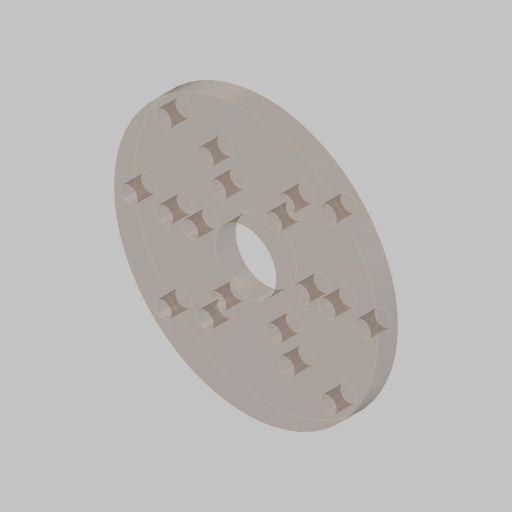
# Autodesk Inventor part: GP9-003
Saved by Autodesk Inventor 2023.5 (Build 275446000, 446)
## iProperties
Created: 2025-02-24
Part Number: GP9-003
Material: Polycarbonate, Smoke
Document SubType Name: Modeling
Designer: dlangdon
Density: 1.2 g/cm^3
Appearance: Polycarbonate - Smoked
Author: dlangdon
Autodesk Inventor part; units mm, degrees
ref_plane "YZ Plane" through (0, 0, 0) normal (1, 0, 0) x (0, 1, 0)
ref_plane "XZ Plane" through (0, 0, 0) normal (0, 1, 0) x (-1, 0, 0)
ref_plane "XY Plane" through (0, 0, 0) normal (0, 0, 1) x (1, 0, 0)
sketch "Sketch1" plane through (0, 0, 0) normal (0, 0, 1) x (1, 0, 0)
  circle A0 centre (0, 0) radius 9.525
  circle A1 centre (0, 0) radius 31.75 construction
  circle A2 centre (-36.5125, 0) radius 4.7625 construction
  circle A3 centre (36.5125, 0) radius 4.7625 construction
  circle A4 centre (0, 0) radius 17.4625 construction
  line L0 (-36.5125, 0) -> (36.5125, 0) construction
  circle A5 centre (0, 0) radius 25.4 construction
  circle A6 centre (0, 0) radius 36.5125 construction
  line L1 (0, 36.5125) -> (0, 0) construction
  line L2 (-25.8182, 25.8182) -> (0, 0) construction
  circle A7 centre (-25.8182, 25.8182) radius 4.7625 construction
  circle A8 centre (-25.8182, -25.8182) radius 4.7625 construction
  circle A9 centre (25.8182, -25.8182) radius 4.7625 construction
  circle A10 centre (25.8182, 25.8182) radius 4.7625 construction
  circle A11 centre (0, 0) radius 41.275
  point P0 (-17.4625, 0)
  point P1 (-25.4, 0)
  point P2 (-12.7, -21.997)
  point P3 (-8.7313, -15.123)
  point P4 (12.7, -21.997)
  point P5 (8.7312, -15.123)
  point P6 (25.4, 0)
  point P7 (17.4625, 0)
  point P8 (12.7, 21.997)
  point P9 (8.7313, 15.123)
  point P10 (-12.7, 21.997)
  point P11 (-8.7312, 15.123)
  dimension "d3" = 34.925
  dimension "d18" = 50.8
  dimension "d0" = 19.05
  dimension "d1" = 63.5
  dimension "d2" = 9.525
  dimension "d21" = 360
  dimension "d30" = 45
  dimension "d33" = 360
  dimension "d37" = 360
  constraints: 12 coincident, 10 centre point, 6 end point, 5 horizontal alignment, 3 point on circle, 2 equal radius, 1 horizontal, 1 midpoint, 1 point on line, 1 tangent, 1 vertical, 31 other
  measures "d0" diameter of A0
  measures "d1" diameter of A1
  measures "d2" diameter of A2
  measures "d30" angle of L1 L2
extrude "Extrusion1" add sketch "Sketch1" along normal blind 6.35
hole "Hole2" at (-17.4625, 0, 0) at (-36.5125, 0, 0) at (36.5125, 0, 0) at (-25.4, 0, 0) at (-12.7, -21.997, 0) at (-8.7313, -15.123, 0) at (12.7, -21.997, 0) at (8.7312, -15.123, 0) at (25.4, 0, 0) at (17.4625, 0, 0) at (12.7, 21.997, 0) at (8.7313, 15.123, 0) at (-12.7, 21.997, 0) at (-8.7312, 15.123, 0) at (-25.8182, 25.8182, 0) at (25.8182, 25.8182, 0) at (25.8182, -25.8182, 0) at (-25.8182, -25.8182, 0) direction (0, 0, 1) diameter 5.1054 end through all clearance for "Flat Head Machine Screw (82)" size "#10" standard "Ansi Unified Screw Threads"
body "Solid1"
